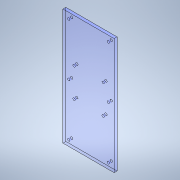
# Autodesk Inventor part: Plaque gauche
Saved by Autodesk Inventor 2022 (Build 260153000, 153)
## iProperties
Created: 2022-05-23
Part Number: Plaque gauche
Material: Générique
Document SubType Name: Modeling
Designer: victo
Density: 1 g/cm^3
Appearance: Transparent - Bleu
Author: victo
Autodesk Inventor part; units mm, degrees
ref_plane "YZ Plane" through (0, 0, 0) normal (1, 0, 0) x (0, 1, 0)
ref_plane "XZ Plane" through (0, 0, 0) normal (0, 1, 0) x (-1, 0, 0)
ref_plane "XY Plane" through (0, 0, 0) normal (0, 0, 1) x (1, 0, 0)
sketch "Esquisse1" plane through (0, 0, 0) normal (0, 0, 1) x (1, 0, 0)
  line L0 (0, 0) -> (-44, 0)
  line L1 (-44, 0) -> (-44, 200)
  line L2 (-44, 200) -> (44, 200)
  line L3 (44, 200) -> (44, 0)
  line L4 (44, 0) -> (0, 0)
  line L5 (-34, 200) -> (-34, 190)
  line L6 (-34, 190) -> (-34, 100) construction
  line L7 (-34, 100) -> (-34, 10) construction
  line L8 (-34, 10) -> (-34, 0)
  line L9 (34, 0) -> (34, 10)
  line L10 (34, 10) -> (34, 100) construction
  line L11 (34, 100) -> (34, 190) construction
  line L12 (34, 190) -> (34, 200)
  circle A0 centre (-34, 190) radius 2
  circle A1 centre (34, 190) radius 2
  circle A2 centre (34, 100) radius 2
  circle A3 centre (-34, 100) radius 2
  circle A4 centre (-34, 10) radius 2
  circle A5 centre (34, 10) radius 2
  line L13 (-34, 10) -> (-44, 10)
  line L14 (34, 10) -> (44, 10)
  line L15 (25, 125) -> (-25, 125) construction
  line L16 (-25, 125) -> (-25, 75) construction
  line L17 (-25, 75) -> (25, 75) construction
  line L18 (25, 75) -> (25, 125) construction
  line L19 (25, 125) -> (-25, 75) construction
  line L20 (-25, 125) -> (25, 75) construction
  line L21 (-34, 100) -> (34, 100) construction
  circle A6 centre (-25, 125) radius 2
  circle A7 centre (25, 125) radius 2
  circle A8 centre (25, 75) radius 2
  circle A9 centre (-25, 75) radius 2
  point P0 (0, 100)
  dimension "d0" = 200
  dimension "d3" = 88
  dimension "d4" = 10
  dimension "d5" = 4
  dimension "d8" = 4
  dimension "d9" = 50
  dimension "d10" = 50
  constraints: 44 end point, 13 point on line, 10 centre point, 10 coincident, 8 equal length, 8 equal radius, 6 perpendicular, 3 midpoint, 2 horizontal, 2 parallel, 2 vertical
  measures "d0" distance between parallel lines of L0 L2
  measures "d3" distance between parallel lines of L1 L3
  measures "d4" distance of L5.start L5.end
  measures "d5" diameter of A3
  measures "d8" diameter of A9
  measures "d9" distance of L15.end L16.end
  measures "d10" distance of L15.start L15.end
extrude "Extrusion1" add sketch "Esquisse1" against normal blind 5 contours L0 L8 A4 L13 L1 L2 L3 L14 A5 L9 L4 | L0 L1 L13 A4 L8 | L9 A5 L14 L3 L4
